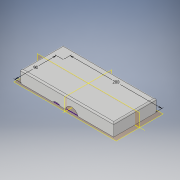
# Autodesk Inventor part: top
Saved by Autodesk Inventor 2019 (Build 230136000, 136)
## iProperties
Created: 2019-08-09
Part Number: top
Material: Generic
Document SubType Name: Modeling
Designer: tmst0
Density: 1 g/cm^3
Appearance: Default
Author: tmst0
Autodesk Inventor part; units mm, degrees
sketch "Sketch8" plane through (0, 0, 0) normal (0, 1, 0) x (-1, 0, 0)
  line L0 (101.5, -46.5) -> (-101.5, -46.5)
  line L1 (-101.5, -46.5) -> (-101.5, 46.5)
  line L2 (-101.5, 46.5) -> (101.5, 46.5)
  line L3 (101.5, 46.5) -> (101.5, -46.5)
  line L4 (101.5, -46.5) -> (-101.5, 46.5) construction
  line L5 (-101.5, -46.5) -> (101.5, 46.5) construction
  point P0 (0, 0)
  dimension "d19" = 203
  dimension "d20" = 93
  constraints: 12 end point, 2 midpoint, 2 parallel, 1 horizontal, 1 perpendicular
  measures "d19" distance of L1.end L2.end
  measures "d20" distance of L0.end L1.end
extrude "Extrusion4" add sketch "Sketch8" along normal blind 26.5
shell "Shell3" thickness 3 removed faces 1 at (-33.8333, 0, 15.5)
sketch "Sketch11" plane through (0, 0, 0) normal (0, 1, 0) x (-1, 0, 0)
  line L0 (-100, 45) -> (100, 45)
  line L1 (100, 45) -> (100, -45)
  line L2 (100, -45) -> (-100, -45)
  line L3 (-100, -45) -> (-100, 45)
  line L4 (-100, 45) -> (100, -45) construction
  line L5 (100, 45) -> (-100, -45) construction
  point P0 (0, 0)
  dimension "d28" = 200
  dimension "d29" = 90
  constraints: 12 end point, 2 midpoint, 2 parallel, 1 horizontal, 1 perpendicular
  measures "d28" distance of L1.end L2.end
  measures "d29" distance of L0.end L1.end
extrude "Extrusion6" cut sketch "Sketch11" along normal blind 5
fillet "Fillet1" radius 3 4 edges at (0, 26.5, 46.5) (101.5, 26.5, 0) (0, 26.5, -46.5) (-101.5, 26.5, 0)
sketch "Sketch13" plane through (-101.5, 0, 46.5) normal (0, 0, 1) x (1, 0, 0)
  circle A0 centre (111.5, -3) radius 14
  circle A1 centre (78.5, -8) radius 11.5
  line L0 (-40.6, 0) -> (243.6, 0) projected
  line L1 (203, 0) -> (203, 23.5) projected
  point P0 (101.5, 0)
  dimension "d74" = 28
  dimension "d75" = 23
  dimension "d76" = 3
  dimension "d77" = 91.5
  dimension "d78" = 124.5
  dimension "d79" = 8
  constraints: 2 centre point
  measures "d74" diameter of A0
  measures "d75" diameter of A1
  measures "d76" distance from line of A0.centre L0
  measures "d77" distance from line of L1 A0.centre
  measures "d78" distance from line of L1 A1.centre
  measures "d79" distance from line of L0 A1.centre
extrude "Extrusion8" cut sketch "Sketch13" against normal blind 10
body "Solid4"
